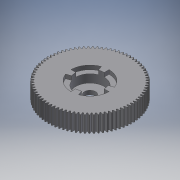
# Autodesk Inventor part: gear 4 clutch
Saved by Autodesk Inventor 2017 (Build 210142000, 142)
## iProperties
Created: 2018-04-17
Part Number: gear 4 clutch
Material: Generic
Document SubType Name: Modeling
Designer: RKL
Density: 1 g/cm^3
Appearance: Default
Author: RKL
Autodesk Inventor part; units mm, degrees
ref_plane "YZ Plane" through (0, 0, 0) normal (1, 0, 0) x (0, 1, 0)
ref_plane "XZ Plane" through (0, 0, 0) normal (0, 1, 0) x (-1, 0, 0)
ref_plane "XY Plane" through (0, 0, 0) normal (0, 0, 1) x (1, 0, 0)
sketch "Sketch1" plane through (0, 0, 0) normal (0, 0, 1) x (1, 0, 0)
  spline S0 degree 3 poles (-1.6094, 51.725) (-1.4848, 51.4472) (-1.2356, 50.8916) (-0.9039, 50.0383) (-0.7246, 49.378) (-0.5898, 48.9796) (-0.5092, 48.8493) (-0.4296, 48.7664) (-0.3355, 48.7006) (-0.1921, 48.6441) (0, 48.6474) (0.1921, 48.6441) (0.3355, 48.7006) (0.4296, 48.7664) (0.5092, 48.8493) (0.5898, 48.9796) (0.7246, 49.378) (0.9039, 50.0383) (1.2356, 50.8916) (1.4848, 51.4472) (1.6094, 51.725) knots 0 0 0 0 0.091359 0.182717 0.27408 0.296885 0.308311 0.319731 0.331128 0.342543 0.365299 0.388056 0.39947 0.410867 0.422287 0.433713 0.456518 0.547881 0.63924 0.730598 0.730598 0.730598 0.730598
  circle A0 centre (0, 0) radius 48.6461 construction
  circle A1 centre (0, 0) radius 47.5719 construction
  circle A2 centre (0, 0) radius 50.625 construction
  circle A3 centre (0, 0) radius 51.75
  point P0 (-1.2426, 50.8883)
  point P1 (-0.9194, 50.0338)
  point P2 (-0.6501, 49.1607)
  point P3 (-0.5671, 48.9483)
  point P4 (-0.506, 48.8517)
  point P5 (-0.4272, 48.7692)
  point P6 (-0.3333, 48.7045)
  point P7 (-0.2269, 48.6631)
  point P8 (0, 48.6461)
  point P9 (0.2269, 48.6631)
  point P10 (0.3333, 48.7045)
  point P11 (0.4272, 48.7692)
  point P12 (0.506, 48.8517)
  point P13 (0.5671, 48.9483)
  point P14 (0.6501, 49.1607)
  point P15 (0.9194, 50.0338)
  point P16 (1.2426, 50.8883)
  constraints: 4 centre point, 2 point on circle, 43 other
extrude "Extrusion1" add sketch "Sketch1" against normal blind 20
extrude "Extrusion2" cut sketch "Sketch1" against normal through all contours A3 S0 picked at (-0.0887, 50.5)
pattern_circular "Circular Pattern1" count 81 over 360 about axis through (0, 0, 0) along (0, 0, -1) of "Extrusion2"
sketch "Sketch2" plane through (0, 0, 0) normal (0, 0, 1) x (1, 0, 0)
  circle A0 centre (0, 0) radius 6.75
  dimension "d7" = 13.5
  constraints: 1 centre point, 1 coincident
  measures "d7" diameter of A0
extrude "Extrusion3" cut sketch "Sketch2" against normal through all
sketch "Sketch3" plane through (0, 0, 0) normal (0, 0, 1) x (1, 0, 0)
  circle A0 centre (0, 0) radius 17.5
  dimension "d10" = 35
  constraints: 1 centre point, 1 coincident
  measures "d10" diameter of A0
extrude "Extrusion4" cut sketch "Sketch3" against normal blind 15
sketch "Sketch4" plane through (0, 0, 0) normal (0, 0, 1) x (1, 0, 0)
  circle A0 centre (0, 0) radius 17.5 construction
  line L0 (0, 0) -> (0, 17.5) construction
  line L1 (0, 17.5) -> (0, 23.5)
  arc A1 (22.0828, 8.0375) -> (0, 23.5) centre (0, 0) ccw
  arc A2 (16.4446, 5.9854) -> (0, 17.5) centre (0, 0) ccw
  line L2 (22.0828, 8.0375) -> (16.4446, 5.9854)
  dimension "d13" = 6
  dimension "d14" = 70
  constraints: 6 end point, 4 point on circle, 2 centre point, 2 coincident, 2 vertical, 1 line through centre, 1 vertical alignment, 1 other
  measures "d13" distance of L0.end L1.end
  measures "d14" angle of L2 L1
extrude "Extrusion5" cut sketch "Sketch4" against normal blind 5
pattern_circular "Circular Pattern2" count 4 over 360 about axis through (0, 0, 0) along (0, 0, -1) of "Extrusion5"
equation "\"d0\" = FaceWidth"
equation "\"Module\" = 1.25"
equation "\"PressureAngle\" = 20deg"
equation "\"UnitProfileClearance\" = 0.25"
equation "\"UnitRoundRadius\" = 0.35"
equation "\"HeadDiameter\" = 103.5"
equation "\"RootDiameter\" = 97.29212"
equation "\"BaseDiameter\" = 95.14388"
equation "\"PitchDiameter\" = 101.25"
equation "\"FaceWidth\" = 20"
equation "\"HelixAngle\" = 0"
equation "\"UnitCorrection\" = -0.099247"
equation "\"UnitAddendumModification\" = 0.000753"
equation "\"CircularPitch\" = 3.926991"
equation "\"UnitBacklashShift\" = -0.233904"
equation "\"TotalToolShift\" = -0.41644"
equation "\"IsInternal\" = 0"
body "Solid1"
